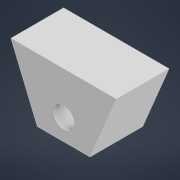
# Autodesk Inventor part: 2
Saved by Autodesk Inventor 2021.2 (Build 252289000, 289)
## iProperties
Created: 2023-09-06
Part Number: 2
Material: Типовые
Document SubType Name: Modeling
Designer: User
Density: 1 g/cm^3
Appearance: По умолчанию
Author: User
Autodesk Inventor part; units mm, degrees
ref_plane "YZ Plane" through (0, 0, 0) normal (1, 0, 0) x (0, 1, 0)
ref_plane "XZ Plane" through (0, 0, 0) normal (0, 1, 0) x (-1, 0, 0)
ref_plane "XY Plane" through (0, 0, 0) normal (0, 0, 1) x (1, 0, 0)
sketch "Эскиз1" plane through (0, 0, 0) normal (0, 0, 1) x (1, 0, 0)
  line L0 (-10, 0) -> (10, 0)
  line L1 (-20, 24) -> (20, 24)
  line L2 (20, 24) -> (10, 0)
  line L3 (-10, 0) -> (-20, 24)
  circle A0 centre (0, 8) radius 4
  line L4 (-20, 24) -> (-20, 30)
  line L5 (-20, 30) -> (20, 30)
  line L6 (20, 30) -> (20, 24)
  line L7 (-5.2413, 8) -> (5.4825, 8)
  point P0 (0, 0)
  dimension "d0" = 20
  dimension "d1" = 40
  dimension "d3" = 8
  dimension "d5" = 24
  dimension "d6" = 6
  dimension "d7" = 16
  constraints: 16 end point, 3 horizontal, 2 perpendicular, 1 centre point, 1 vertical
  measures "d0" distance of L0.start L0.end
  measures "d1" distance of L1.start L1.end
  measures "d3" diameter of A0
  measures "d5" vertical distance of L0.start L1.start
  measures "d6" distance of L1.start L4.end
  measures "d7" distance from line of L1 L7.end
extrude "Выдавливание1" add sketch "Эскиз1" along normal mid plane 20 contours L3 L1 L2 L0
